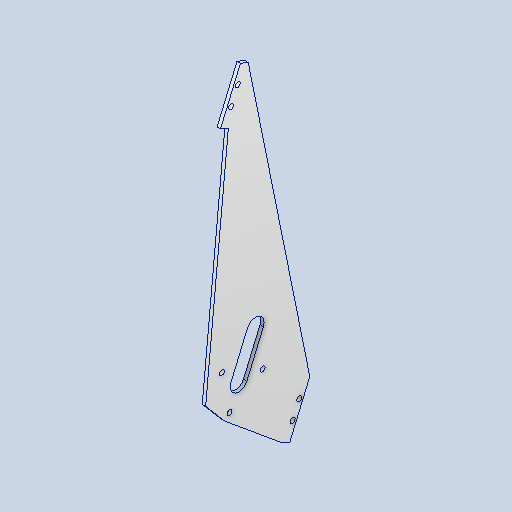
# Autodesk Inventor part: belt_liner_v2_Plate_2
Saved by Autodesk Inventor 2025.2 (Build 292293000, 293)
## iProperties
Created: 2025-01-05
Part Number: belt_liner_v2_Plate_2
Material: アルミニウム 6061
Document SubType Name: Modeling
Designer: haruy
Density: 2.7 g/cm^3
Appearance: アルミニウム - フラット
Author: haruy
Autodesk Inventor part; units mm, degrees
ref_plane "YZ Plane" through (0, 0, 0) normal (1, 0, 0) x (0, 1, 0)
ref_plane "XZ Plane" through (0, 0, 0) normal (0, 1, 0) x (-1, 0, 0)
ref_plane "XY Plane" through (0, 0, 0) normal (0, 0, 1) x (1, 0, 0)
derived "belt_liner_v2_Sketch_Base.ipt"
sketch "スケッチ1" plane through (300, 0, 0) normal (1, 0, 0) x (0, 1, 0)
  circle A0 centre (0, 0) radius 23.875
  circle A1 centre (981.9946, -416.832) radius 23.875 construction
  line L0 (0, 0) -> (0, -985.832)
  line L1 (0.8886, 67.5475) -> (6.7495, 81.3551)
  line L2 (6.7495, 81.3551) -> (503.8221, -129.6397)
  line L3 (503.8221, -129.6397) -> (497.9612, -143.4473)
  line L4 (497.9612, -143.4473) -> (0.8886, 67.5475)
  line L5 (0, 0) -> (981.9946, -416.832)
  line L6 (-41.3299, -31.913) -> (-47.1909, -45.7206)
  line L7 (-47.1909, -45.7206) -> (953.3979, -470.4453)
  line L8 (953.3979, -470.4453) -> (959.2588, -456.6378)
  line L9 (959.2588, -456.6378) -> (-41.3299, -31.913)
  line L10 (11.023, 79.5411) -> (11.023, 79.5411)
  line L11 (0.8886, 67.5475) -> (82.443, 32.9297)
  line L12 (82.443, 32.9297) -> (80.4894, 28.3272)
  line L13 (80.4894, 28.3272) -> (-1.0651, 62.945)
  line L14 (-1.0651, 62.945) -> (0.8886, 67.5475)
  line L15 (497.9612, -143.4473) -> (479.78, -135.7298)
  line L16 (0, -985.832) -> (0, 0)
  circle A2 centre (0, 0) radius 12.5
  circle A3 centre (0, 0) radius 15
  line L17 (0, 0) -> (0, 0)
  circle A4 centre (0, 0) radius 25.575 construction
  line L18 (0, 0) -> (0, 0)
  line L19 (0, 0) -> (0, 0)
  line L20 (-41.3299, -31.913) -> (-39.3763, -27.3105)
  line L21 (-39.3763, -27.3105) -> (35.0455, -58.9007)
  line L22 (39.5354, -66.2383) -> (-41.3299, -31.913)
  line L23 (84.9924, 48.1429) -> (503.8221, -129.6397)
  line L24 (503.8221, -129.6397) -> (505.9712, -124.5769)
  circle A5 centre (981.9946, -416.832) radius 5
  line L25 (959.2588, -456.6378) -> (931.6437, -444.9158)
  line L26 (931.6437, -444.9158) -> (933.5973, -440.3133)
  line L27 (933.5973, -440.3133) -> (961.2125, -452.0352)
  line L28 (961.2125, -452.0352) -> (959.2588, -456.6378)
  circle A6 centre (977.3921, -414.8783) radius 5.1
  line L29 (981.9946, -416.832) -> (543.1871, -230.5692)
  circle A7 centre (1000.4047, -424.6466) radius 5.1
  line L30 (979.3848, -410.1837) -> (1002.3974, -419.952)
  line L31 (975.3993, -419.5729) -> (998.4119, -429.3412)
  circle A8 centre (981.9946, -416.832) radius 22.175 construction
  line L32 (1033.1157, -370.6069) -> (1016.705, -409.2681)
  line L33 (1016.705, -409.2681) -> (1025.9101, -413.1754)
  line L34 (1025.9101, -413.1754) -> (1042.3208, -374.5142)
  line L35 (1042.3208, -374.5142) -> (1033.1157, -370.6069)
  circle A9 centre (977.3921, -414.8783) radius 10.1 construction
  circle A10 centre (1000.4047, -424.6466) radius 10.1 construction
  line L36 (981.3384, -405.5812) -> (1004.3511, -415.3495) construction
  line L37 (973.4457, -424.1754) -> (996.4583, -433.9437) construction
  line L38 (981.3384, -405.5812) -> (970.227, -400.8647) construction
  line L39 (968.095, -410.9319) -> (972.0413, -401.6348) construction
  line L40 (1004.3511, -415.3495) -> (1013.1977, -419.1047) construction
  line L41 (1013.1977, -419.1047) -> (1013.5561, -419.2568)
  line L42 (82.443, 32.9297) -> (80.4894, 28.3272)
  line L43 (80.4894, 28.3272) -> (103.4122, 18.597)
  line L44 (103.4122, 18.597) -> (105.3659, 23.1995)
  line L45 (105.3659, 23.1995) -> (82.443, 32.9297)
  line L46 (-47.1909, -45.7206) -> (-47.1909, -625.2553)
  line L47 (996.4583, -433.9437) -> (1004.3511, -415.3495)
  line L48 (1004.3511, -415.3495) -> (1013.5561, -419.2568)
  line L49 (1013.5561, -419.2568) -> (1005.6633, -437.851)
  line L50 (1005.6633, -437.851) -> (996.4583, -433.9437) construction
  line L51 (503.8221, -129.6397) -> (497.9612, -143.4473)
  line L52 (497.9612, -143.4473) -> (1139.5531, -415.7869)
  line L53 (1139.5531, -415.7869) -> (1145.414, -401.9793)
  line L54 (1145.414, -401.9793) -> (503.8221, -129.6397)
  line L55 (-12.3385, -2.003) -> (-33.3833, -51.5816)
  line L56 (-12.3385, -2.003) -> (20.5571, 75.4941)
  circle A11 centre (36.7319, 49.617) radius 1.5
  circle A12 centre (59.7445, 39.8487) radius 1.5
  circle A13 centre (951.0306, -450.4292) radius 1.5
  circle A14 centre (0, 0) radius 45
  circle A15 centre (59.8757, 3.8601) radius 22 construction
  circle A16 centre (59.8757, 3.8601) radius 15
  circle A17 centre (92.9223, 14.3588) radius 3
  circle A18 centre (50.8799, -21.5972) radius 3
  circle A19 centre (50.8799, -21.5972) radius 4 construction
  circle A20 centre (38.8164, -45.7524) radius 22 construction
  circle A21 centre (38.8164, -45.7524) radius 15
  circle A22 centre (50.8799, -21.5972) radius 3
  line L57 (63.1278, -76.307) -> (65.0815, -71.7045)
  line L58 (103.4122, 18.597) -> (65.0815, -71.7045)
  circle A23 centre (82.7572, 30.0805) radius 1.5
  circle A24 centre (981.9946, -416.832) radius 6 construction
  circle A25 centre (0, 0) radius 25.575 construction
  circle A26 centre (0, 0) radius 25.525
  circle A27 centre (981.9946, -416.832) radius 25.525
  line L59 (991.968, -393.3361) -> (9.9734, 23.4959)
  circle A28 centre (964.4129, -409.369) radius 4
  circle A29 centre (964.4129, -409.369) radius 1.5
  circle A30 centre (981.9946, -416.832) radius 18.525 construction
  circle A31 centre (987.1661, -404.9045) radius 4
  line L60 (978.1402, -426.1681) -> (982.0866, -416.871)
  circle A32 centre (987.1661, -404.9045) radius 1.5
  line L61 (972.0413, -401.6348) -> (974.7374, -395.2833) construction
  line L62 (974.7374, -395.2833) -> (1016.2522, -412.9053)
  line L63 (1013.5561, -419.2568) -> (1016.2522, -412.9053)
  line L64 (974.7374, -395.2833) -> (961.8141, -406.3282)
  line L65 (961.4525, -426.5805) -> (1002.9673, -444.2025)
  line L66 (961.4525, -426.5805) -> (960.4203, -409.6119)
  line L67 (1005.6633, -437.851) -> (1002.9673, -444.2025)
  circle A33 centre (977.0071, -428.8376) radius 4
  circle A34 centre (977.0071, -428.8376) radius 1.5
  circle A35 centre (294.227, 105.9868) radius 120
  line L68 (111.9353, -6.7481) -> (102.7303, -2.8408) construction
  line L69 (1139.5531, -415.7869) -> (1111.9379, -404.065)
  line L70 (1111.9379, -404.065) -> (1109.9843, -408.6675)
  line L71 (1109.9843, -408.6675) -> (1137.5994, -420.3894)
  line L72 (1137.5994, -420.3894) -> (1139.5531, -415.7869)
  circle A36 centre (1129.3712, -414.1808) radius 1.5
  line L73 (103.4122, 18.597) -> (105.3659, 23.1995)
  line L74 (105.3659, 23.1995) -> (115.9517, 18.7061)
  line L75 (115.9517, 18.7061) -> (113.998, 14.1036)
  line L76 (113.998, 14.1036) -> (103.4122, 18.597)
  circle A37 centre (1120.1661, -410.2735) radius 1.5
  circle A38 centre (941.8256, -446.5219) radius 1.5
  line L77 (35.0455, -58.9007) -> (65.101, -71.6585)
  line L78 (503.8221, -129.6397) -> (505.9712, -124.5769)
  line L79 (122.5941, 34.3547) -> (184.7282, 7.9804)
  line L80 (184.7282, 7.9804) -> (186.6818, 12.5829)
  line L81 (186.6818, 12.5829) -> (124.5477, 38.9572)
  line L82 (124.5477, 38.9572) -> (122.5941, 34.3547)
  circle A39 centre (136.6965, 38.1458) radius 4
  circle A40 centre (136.6965, 38.1458) radius 11
  circle A41 centre (164.3116, 26.4239) radius 4
  circle A42 centre (164.3116, 26.4239) radius 11
  line L83 (134.5175, 22.7753) -> (131.7824, 16.3318)
  line L84 (131.7824, 16.3318) -> (152.0335, 7.7357)
  line L85 (152.0335, 7.7357) -> (154.7686, 14.1793)
  line L86 (154.7686, 14.1793) -> (134.5175, 22.7753)
  line L87 (144.6431, 18.4773) -> (141.908, 12.0338)
  line L88 (162.1327, 11.0534) -> (159.3976, 4.6099)
  line L89 (159.3976, 4.6099) -> (179.6487, -3.9862)
  line L90 (179.6487, -3.9862) -> (182.3838, 2.4573)
  line L91 (182.3838, 2.4573) -> (162.1327, 11.0534)
  line L92 (172.2582, 6.7554) -> (169.5231, 0.3118)
  line L93 (3.819, 74.4513) -> (1142.4835, -408.8831)
  line L94 (177.3043, -9.5092) -> (175.3506, -14.1118)
  line L95 (115.1702, 16.8651) -> (177.3043, -9.5092)
  line L96 (175.3506, -14.1118) -> (113.2165, 12.2626)
  line L97 (113.2165, 12.2626) -> (115.1702, 16.8651)
  circle A43 centre (122.2394, 4.0872) radius 11
  circle A44 centre (122.2394, 4.0872) radius 4
  circle A45 centre (149.8546, -7.6348) radius 11
  circle A46 centre (149.8546, -7.6348) radius 4
  line L98 (143.3054, 25.5633) -> (150.6695, 22.4374)
  line L99 (150.6695, 22.4374) -> (143.2456, 4.9478)
  line L100 (143.2456, 4.9478) -> (135.8816, 8.0737)
  line L101 (135.8816, 8.0737) -> (143.3054, 25.5633)
  line L102 (170.9206, 13.8413) -> (178.2846, 10.7155)
  line L103 (178.2846, 10.7155) -> (170.8607, -6.7741)
  line L104 (170.8607, -6.7741) -> (163.4967, -3.6483)
  line L105 (163.4967, -3.6483) -> (170.9206, 13.8413)
  line L106 (113.2165, 12.2626) -> (99.541, -19.9551)
  line L107 (99.541, -19.9551) -> (108.746, -23.8624)
  line L108 (108.746, -23.8624) -> (122.4216, 8.3553)
  line L109 (122.4216, 8.3553) -> (113.2165, 12.2626)
  line L110 (113.2165, 12.2626) -> (150.9572, -3.7574)
  line L111 (150.9572, -3.7574) -> (147.8314, -11.1214)
  line L112 (147.8314, -11.1214) -> (110.0907, 4.8986)
  line L113 (110.0907, 4.8986) -> (113.2165, 12.2626)
  line L114 (133.9279, 3.4711) -> (141.2919, 0.3453)
  line L115 (141.2919, 0.3453) -> (140.1197, -2.4162)
  line L116 (140.1197, -2.4162) -> (132.7557, 0.7096)
  line L117 (132.7557, 0.7096) -> (133.9279, 3.4711)
  circle A47 centre (60.8628, -61.1686) radius 3
  circle A48 centre (-3.5329, -45.241) radius 1.25
  circle A49 centre (19.4797, -55.0093) radius 1.25
  circle A50 centre (42.4923, -64.7776) radius 1.25
  circle A51 centre (294.227, 105.9868) radius 130
  line L118 (294.227, 105.9868) -> (183.7664, 152.8745)
  line L119 (294.227, 105.9868) -> (182.9649, 61.034)
  line L120 (294.227, 105.9868) -> (249.2742, 217.2489)
  line L121 (251.6186, 222.7719) -> (180.6205, 55.511)
  line L122 (180.6205, 55.511) -> (175.0975, 57.8554)
  line L123 (175.0975, 57.8554) -> (246.0955, 225.1163)
  line L124 (246.0955, 225.1163) -> (251.6186, 222.7719)
  line L125 (294.227, 105.9868) -> (243.4319, -13.6788)
  line L126 (1032.3343, -372.4479) -> (1030.3806, -377.0505)
  line L127 (1030.3806, -377.0505) -> (1092.5147, -403.4248)
  line L128 (1092.5147, -403.4248) -> (1094.4683, -398.8223)
  line L129 (1094.4683, -398.8223) -> (1032.3343, -372.4479)
  line L130 (1094.4683, -398.8223) -> (1092.5147, -403.4248)
  line L131 (1092.5147, -403.4248) -> (1109.2028, -410.5085)
  line L132 (1109.2028, -410.5085) -> (1111.1564, -405.906)
  line L133 (1111.1564, -405.906) -> (1094.4683, -398.8223)
  line L134 (974.7374, -395.2833) -> (1109.9843, -408.6675)
  circle A52 centre (981.9946, -416.832) radius 35.525
  line L135 (1103.3095, -408.0069) -> (1106.0446, -401.5634)
  circle A53 centre (982.0866, -416.871) radius 8.5
  line L136 (221.0764, 266.3645) -> (113.2165, 12.2626)
  line L137 (256.7074, -7.9969) -> (252.7875, -17.2316)
  line L138 (252.7875, -17.2316) -> (175.3506, -14.1118)
  line L139 (180.6205, 55.511) -> (201.0962, 30.3121)
  line L140 (246.0955, 225.1163) -> (246.9277, 227.0768)
  circle A54 centre (128.1734, 34.7023) radius 1.5
  circle A55 centre (181.1025, 12.2353) radius 1.5
  circle A56 centre (118.7959, 12.6102) radius 1.5
  circle A57 centre (171.7249, -9.8568) radius 1.5
  line L141 (175.0975, 57.8554) -> (177.4419, 63.3784)
  line L142 (177.4419, 63.3784) -> (172.8393, 65.3321)
  line L143 (172.8393, 65.3321) -> (170.495, 59.809)
  line L144 (170.495, 59.809) -> (175.0975, 57.8554)
  line L145 (246.0955, 225.1163) -> (243.7511, 219.5933)
  line L146 (243.7511, 219.5933) -> (239.1486, 221.5469)
  line L147 (239.1486, 221.5469) -> (241.493, 227.0699)
  line L148 (241.493, 227.0699) -> (246.0955, 225.1163)
  circle A58 centre (242.6221, 223.3316) radius 1.5
  line L149 (246.9277, 227.0768) -> (241.493, 227.0699)
  line L150 (241.493, 227.0699) -> (222.1215, 214.1571)
  circle A59 centre (173.9684, 61.5937) radius 1.5
  line L151 (1137.5994, -420.3894) -> (959.2588, -456.6378)
  line L152 (933.5973, -440.3133) -> (961.332, -406.8179)
  line L153 (1111.9379, -404.065) -> (1109.9843, -408.6675)
  line L154 (1109.9843, -408.6675) -> (1102.6202, -405.5416)
  line L155 (1102.6202, -405.5416) -> (1104.5739, -400.9391)
  line L156 (1104.5739, -400.9391) -> (1111.9379, -404.065)
  line L157 (-29.8566, -31.7473) -> (-44.8566, -31.7473)
  line L158 (-44.8566, -31.7473) -> (-44.8566, -284.2473)
  line L159 (-44.8566, -284.2473) -> (-29.8566, -284.2473)
  line L160 (-29.8566, -284.2473) -> (-29.8566, -31.7473)
  line L161 (471.1434, -269.2473) -> (-44.8566, -269.2473)
  line L162 (-44.8566, -269.2473) -> (-44.8566, -284.2473)
  line L163 (-44.8566, -284.2473) -> (471.1434, -284.2473)
  line L164 (471.1434, -284.2473) -> (471.1434, -269.2473)
  line L165 (-14.9732, -59.3962) -> (-9.1123, -45.5886)
  line L166 (12.6419, -71.1181) -> (18.5029, -57.3106)
  line L167 (-44.8566, -78.7473) -> (-67.8566, -78.7473)
  line L168 (-67.8566, -78.7473) -> (-67.8566, -138.7473)
  line L169 (-67.8566, -138.7473) -> (-44.8566, -138.7473)
  line L170 (-44.8566, -138.7473) -> (-44.8566, -78.7473)
  line L171 (-44.8566, -98.7473) -> (-89.8566, -98.7473)
  line L172 (-89.8566, -98.7473) -> (-89.8566, -118.7473)
  line L173 (-89.8566, -118.7473) -> (-44.8566, -118.7473)
  line L174 (-44.8566, -118.7473) -> (-44.8566, -98.7473)
  line L175 (-29.8566, -78.7473) -> (-44.8566, -78.7473)
  line L176 (-89.8566, -108.7473) -> (-44.8566, -108.7473)
  line L177 (-53.8566, -248.7473) -> (-58.8566, -248.7473)
  line L178 (-58.8566, -248.7473) -> (-58.8566, -258.7473)
  line L179 (-58.8566, -258.7473) -> (-53.8566, -258.7473)
  line L180 (-53.8566, -258.7473) -> (-53.8566, -248.7473)
  line L181 (-44.8566, -240.249) -> (-49.8566, -240.249)
  line L182 (-49.8566, -240.249) -> (-49.8566, -266.157)
  line L183 (-49.8566, -266.157) -> (-44.8566, -266.157)
  line L184 (-44.8566, -266.157) -> (-44.8566, -240.249)
  line L185 (-47.3566, -240.249) -> (-47.3566, -266.157)
  line L186 (441.1434, -269.2473) -> (441.1434, -284.2473)
  line L187 (471.1434, -284.2473) -> (514.7428, -284.2473)
  line L188 (514.7428, -284.2473) -> (520.6037, -270.4397)
  line L189 (471.1434, -269.2473) -> (479.405, -269.2473)
  line L190 (479.405, -269.2473) -> (485.266, -255.4397)
  line L191 (-58.8566, -253.7473) -> (-53.8566, -253.7473)
  line L192 (-85.8566, 246.1124) -> (-105.8566, 246.1124)
  line L193 (-105.8566, 246.1124) -> (-105.8566, -703.7066)
  line L194 (-105.8566, -703.7066) -> (-85.8566, -703.7066)
  line L195 (-85.8566, -703.7066) -> (-85.8566, 246.1124)
  line L196 (242.6221, 223.3316) -> (-85.8566, 223.3316)
  line L197 (-23.792, -270.0272) -> (-25.5939, -279.8636)
  line L198 (-25.5939, -279.8636) -> (928.4435, -454.6324)
  line L199 (928.4435, -454.6324) -> (930.2454, -444.7961)
  line L200 (930.2454, -444.7961) -> (-23.792, -270.0272)
  point P0 (50.8799, -21.5972)
  point P1 (81.4662, 30.6284)
  point P2 (961.1401, -407.0693)
  point P3 (960.7309, -407.8061)
  point P4 (960.5703, -407.7379)
  point P5 (-27.5224, -37.774)
  point P6 (-37.3566, -41.7473)
  point P7 (-37.3566, -276.7473)
  point P8 (461.1434, -276.7473)
  point P9 (451.1434, -276.7473)
  point P10 (491.9336, -266.4177)
  point P11 (501.1387, -270.325)
  point P12 (-14.8566, -276.7473)
  point P13 (919.5082, -447.9123)
extrude "押し出し2" add sketch "スケッチ1" against normal blind 2 contours L152 A27 L65 L67 L49 L63 L62 L134 A52 L151 | A52 L151 L28 L27 L152 | L5 A28 L66 L65 A27 L152 | L134 L32 A52 | L27 L28 L9 L26 | A28 L5 A29 | L5 A29 A28 | A27 L62 L134 | L65 A33 L60 A53 L31 A7 L47 L48 A27 | A27 L48 L41 L49 L67 L65 | L134 L34 L33 L32 | L33 L34 L134 L131 L132 L71 L151 A52 | A28 L5 A6 A53 L60 A33 L65 L66 | A31 | L64 L62 A27 L48 L47 L30 A53 A6 L5 A28 | L62 L63 L41 L48 A27 | A33 | L71 L70 L52 L72 | L134 L132 L131 | A53 A6 L31 L60 | L60 L31 A53 | A53 L30 A6
